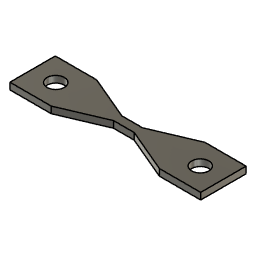
probeta v2 (Autodesk Fusion 360 design; units mm, degrees)
Autodesk Fusion 360 part; units mm, degrees
sketch "Boceto1" plane through (0, 0, 0) normal (0, 0, 1) x (1, 0, 0)
  line L0 (-23.1, 5.5) -> (-23.1, -5.5)
  line L1 (-23.1, -5.5) -> (-13.1, -5.5)
  line L2 (-13.1, -5.5) -> (-2.5, -1)
  line L3 (-2.5, -1) -> (2.5, -1)
  line L4 (2.5, -1) -> (13.1, -5.5)
  line L5 (13.1, -5.5) -> (23.1, -5.5)
  line L6 (23.1, -5.5) -> (23.1, 5.5)
  line L7 (23.1, 5.5) -> (13.1, 5.5)
  line L8 (13.1, 5.5) -> (2.5, 1)
  line L9 (2.5, 1) -> (-2.5, 1)
  line L10 (-2.5, 1) -> (-13.1, 5.5)
  line L11 (-13.1, 5.5) -> (-23.1, 5.5)
  line L12 (0, -1) -> (0, 1) construction
  line L13 (-23.1, 0) -> (23.1, 0) construction
  circle A0 centre (-17.5, 0) radius 2.1
  circle A1 centre (17.5, 0) radius 2.1
  point P0 (-19.6, 0)
  point P1 (-17.5, -2.1)
  dimension "d1" = 11
  dimension "d2" = 4.2
  dimension "d3" = 5
  dimension "d4" = 3.5
  dimension "d5" = 35
  dimension "d6" = 2
  dimension "d7" = 10
  dimension "d8" = 3.4
  constraint vertical L0
  constraint perpendicular L0 L1
  constraint perpendicular L0 L3
  constraint perpendicular L0 L5
  constraint perpendicular L5 L6
  constraint perpendicular L6 L7
  constraint perpendicular L6 L9
  constraint perpendicular L0 L11
  constraint midpoint L3 L12.start
  constraint coincident L9 L12.end
  constraint perpendicular L9 L12
  constraint midpoint origin L12
  constraint equal L0 L6
  constraint equal L1 L5
  constraint symmetric L7.end L10.end L12
  constraint symmetric L0.end L5.end L12
  constraint midpoint L0 L13.start
  constraint midpoint L6 L13.end
  constraint horizontal origin L13.start
  constraint equal L2 L10
  constraint equal L3 L9
  constraint equal L4 L8
  constraint coincident L13 A0.centre
  constraint coincident L13 A1.centre
  constraint symmetric L12 A0.centre A1.centre
  constraint equal A0 A1
  constraint midpoint L9 L12.end
  constraint coincident A0 P0
  constraint coincident L13 P0
  constraint equal L1 L11
  constraint coincident A0 P1
  constraint vertical A0.centre P1
  measures "d1" distance of L0.start L0.end
  measures "d2" diameter of A0
  measures "d3" distance of L2.end L3.end
  measures "d4" distance of L13.start P0
  measures "d5" distance of A0.centre A1.centre
  measures "d6" distance of L3 L9
  measures "d7" distance of L0.start L10.end
  measures "d8" distance of L1 P1
extrude "Extruir1" add sketch "Boceto1" along normal blind 1.6
